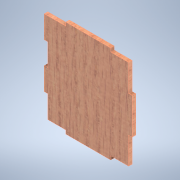
# Autodesk Inventor part: CarSide_V1
Saved by Autodesk Inventor 2022.2 (Build 262287000, 287)
## iProperties
Created: 2022-11-22
Part Number: CarSide_V1
Material: Wood (Oak)
Document SubType Name: Modeling
Designer: jaege
Density: 0.76 g/cm^3
Appearance: Red Oak - Natural Low Gloss
Author: jaege
Autodesk Inventor part; units mm, degrees
ref_plane "YZ Plane" through (0, 0, 0) normal (1, 0, 0) x (0, 1, 0)
ref_plane "XZ Plane" through (0, 0, 0) normal (0, 1, 0) x (-1, 0, 0)
ref_plane "XY Plane" through (0, 0, 0) normal (0, 0, 1) x (1, 0, 0)
sketch "Sketch1" plane through (0, 0, 0) normal (0, 0, 1) x (1, 0, 0)
  line L0 (45, -50) -> (25, -50)
  line L1 (-45, -50) -> (-45, 50)
  line L2 (-45, 50) -> (-25, 50)
  line L3 (45, 50) -> (45, -50)
  line L4 (45, -50) -> (-45, 50) construction
  line L5 (-45, -50) -> (45, 50) construction
  line L6 (-25, 50) -> (25, 50) construction
  line L7 (25, 50) -> (25, 54)
  line L8 (25, 54) -> (-25, 54)
  line L9 (-25, 54) -> (-25, 50)
  line L10 (-25, -50) -> (25, -50) construction
  line L11 (25, -50) -> (25, -54)
  line L12 (25, -54) -> (-25, -54)
  line L13 (-25, -54) -> (-25, -50)
  line L14 (-45, 50) -> (-49, 50)
  line L15 (-49, 50) -> (-49, 25)
  line L16 (-49, 25) -> (-45, 25)
  line L17 (-45, 25) -> (-45, 50)
  line L18 (-45, 0) -> (-45, 25)
  line L19 (-45, 25) -> (-49, 25)
  line L20 (-49, 25) -> (-49, 0)
  line L21 (-49, 0) -> (-45, 0)
  line L22 (-45, -25) -> (-45, 0) construction
  line L23 (-45, 0) -> (-49, 0)
  line L24 (-49, 0) -> (-49, -25)
  line L25 (-49, -25) -> (-45, -25)
  line L26 (-45, -50) -> (-45, -25)
  line L27 (-45, -25) -> (-49, -25)
  line L28 (-49, -25) -> (-49, -50)
  line L29 (-49, -50) -> (-45, -50)
  line L30 (0, -75.6) -> (0, 75.6) projected
  line L31 (45, 20) -> (49, 20)
  line L32 (49, 20) -> (49, -20)
  line L33 (49, -20) -> (45, -20)
  line L34 (45, -20) -> (45, 20)
  line L35 (25, 50) -> (45, 50)
  line L36 (-25, 50) -> (25, 50) construction
  line L37 (-25, -50) -> (-45, -50)
  line L38 (25, -50) -> (-25, -50)
  line L39 (-68.6, 0) -> (68.6, 0) projected
  point P0 (0, 0)
  dimension "d0" = 90
  dimension "d1" = 100
  dimension "d2" = 50
  dimension "d3" = 4
  dimension "d4" = 50
  dimension "d5" = 4
  dimension "d6" = 4
  dimension "d7" = 25
  dimension "d10" = 25
  dimension "d17" = 4
  dimension "d18" = 40
  constraints: 76 end point, 18 parallel, 7 horizontal, 7 perpendicular, 2 midpoint, 1 point on line, 1 symmetric about line, 1 vertical, 1 vertical alignment, 25 other
  measures "d0" distance of L1.end L3.start
  measures "d1" distance of L1.start L1.end
  measures "d2" distance of L8.end L7.end
  measures "d3" distance of L7.end L6.end
  measures "d4" distance of L11.end L12.end
  measures "d5" distance of L0.end L11.end
  measures "d6" distance of L16.end L15.end
  measures "d7" distance of L15.end L14.end
  measures "d10" distance of L16.end L18.start
  measures "d17" distance of L31.start L31.end
  measures "d18" distance of L31.end L32.end
extrude "Extrusion1" add sketch "Sketch1" along normal blind 4 contours L0 L38 L30 L39 L3 | L11 L12 L30 L38 | L3 L39 L32 L33 | L38 L37 L1 L39 L30 | L30 L12 L13 L38 | L39 L30 L8 L7 L35 L3 | L3 L31 L32 L39 | L39 L1 L2 L9 L8 L30 | L1 L25 L24 L21 | L16 L15 L14 L1
body "Solid1"
